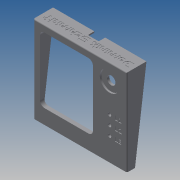
# Autodesk Inventor part: Top
Saved by Autodesk Inventor 2019 (Build 230136000, 136)
## iProperties
Created: 2022-10-27
Part Number: Top
Material: Generisch
Document SubType Name: Modeling
Designer: Dominik Schmidt
Density: 1 g/cm^3
Appearance: Vorgabe
Author: Dominik Schmidt
Autodesk Inventor part; units mm, degrees
ref_plane "YZ Plane" through (0, 0, 0) normal (1, 0, 0) x (0, 1, 0)
ref_plane "XZ Plane" through (0, 0, 0) normal (0, 1, 0) x (-1, 0, 0)
ref_plane "XY Plane" through (0, 0, 0) normal (0, 0, 1) x (1, 0, 0)
sketch "Skizze1" plane through (0, 0, 0) normal (0, 0, 1) x (1, 0, 0)
  line L0 (-19.1, 28.5) -> (19.1, 28.5)
  line L1 (23.1, 24.5) -> (23.1, -24.5)
  line L2 (19.1, -28.5) -> (-19.1, -28.5)
  line L3 (-23.1, -24.5) -> (-23.1, 24.5)
  line L4 (-23.1, 28.5) -> (23.1, -28.5) construction
  line L5 (23.1, 28.5) -> (-23.1, -28.5) construction
  circle A0 centre (37.5, 20) radius 3.7
  arc A1 (-19.1, 28.5) -> (-23.1, 24.5) centre (-19.1, 24.5) ccw
  arc A2 (23.1, 24.5) -> (19.1, 28.5) centre (19.1, 24.5) ccw
  arc A3 (-23.1, -24.5) -> (-19.1, -28.5) centre (-19.1, -24.5) ccw
  arc A4 (19.1, -28.5) -> (23.1, -24.5) centre (19.1, -24.5) ccw
  circle A5 centre (37.5, 20) radius 12
  line L6 (31.4, 28) -> (43.6, 28)
  line L7 (43.6, 28) -> (43.6, 12)
  line L8 (43.6, 12) -> (31.4, 12)
  line L9 (31.4, 12) -> (31.4, 28)
  line L10 (31.4, 28) -> (43.6, 12) construction
  line L11 (43.6, 28) -> (31.4, 12) construction
  line L12 (-25.5, 32) -> (25.5, 32)
  line L13 (25.5, 32) -> (25.5, -32)
  line L14 (25.5, -32) -> (-25.5, -32)
  line L15 (-25.5, -32) -> (-25.5, 32)
  line L16 (-25.5, 32) -> (25.5, -32) construction
  line L17 (25.5, 32) -> (-25.5, -32) construction
  circle A6 centre (37.5, -5) radius 1.5
  circle A7 centre (37.5, -13) radius 1.5
  circle A8 centre (37.5, -21) radius 1.5
  line L18 (-27.5, 33) -> (51.5, 33)
  line L19 (51.5, 33) -> (51.5, -33)
  line L20 (-27.5, -33) -> (-27.5, 33)
  line L21 (52.7, 34.2) -> (-28.7, 34.2)
  line L22 (-28.7, 34.2) -> (-28.7, -34.2)
  line L23 (52.7, -34.2) -> (52.7, 34.2)
  line L24 (-27.72, -34.2) -> (-27.2531, -34.2)
  line L25 (52.7, -34.2) -> (52.7, -41.2)
  line L26 (52.7, -41.2) -> (-28.7, -41.2)
  line L27 (-28.7, -41.2) -> (-28.7, -34.2)
  line L28 (-27.5, -33) -> (-27.5, -40)
  line L29 (-27.5, -40) -> (51.5, -40)
  line L30 (51.5, -40) -> (51.5, -33)
  point P0 (0, 0)
  dimension "d3" = 57
  dimension "d4" = 46.2
  dimension "d5" = 4
  dimension "d6" = 4
  dimension "d7" = 7.4
  dimension "d8" = 24
  dimension "d9" = 12.2
  dimension "d10" = 16
  dimension "d11" = 51
  dimension "d12" = 64
  dimension "d13" = 12
  dimension "d14" = 12
  dimension "d15" = 3
  dimension "d16" = 3
  dimension "d17" = 3
  dimension "d18" = 5
  dimension "d19" = 8
  dimension "d20" = 8
  dimension "d21" = 2
  dimension "d22" = 1
  dimension "d24" = 14
  dimension "d25" = 1.2
  dimension "d66" = 7
  dimension "d67" = 7
  constraints: 62 end point, 10 parallel, 10 point on line, 9 centre point, 9 perpendicular, 8 point on circle, 8 tangent, 6 midpoint, 4 horizontal, 2 equal radius, 1 coincident, 1 vertical, 1 other
  measures "d3" distance of L5.end L4.start
  measures "d4" distance of L4.start L5.start
  measures "d5" radius of A1
  measures "d6" radius of A2
  measures "d7" diameter of A0
  measures "d8" diameter of A5
  measures "d9" distance of L7.end L8.end
  measures "d10" distance of L6.end L7.end
  measures "d11" distance of L13.end L14.end
  measures "d12" distance of L12.end L13.end
  measures "d13" distance from line of L13 A0.centre
  measures "d14" distance from line of L12 A0.centre
  measures "d15" diameter of A6
  measures "d16" diameter of A7
  measures "d17" diameter of A8
  measures "d18" vertical distance of A6.centre point (0, 0)
  measures "d19" distance of A7.centre A6.centre
  measures "d20" distance of A8.centre A7.centre
  measures "d21" distance between parallel lines of L20 L15
  measures "d22" distance between parallel lines of L12 L18
  measures "d24" distance from line of L19 A0.centre
  measures "d25" distance between parallel lines of L18 L21
  measures "d66" distance of L23.start L25.end
  measures "d67" distance of L20.start L28.end
extrude "Extrusion1" add sketch "Skizze1" along normal blind 3.5 contours L13 L14 L15 L12
extrude "Extrusion2" add sketch "Skizze1" along normal blind 3.5 contours A5 | L6 L7 L8 L9 | L18 L19 L30 L29 L28 L20
extrude "Extrusion3" add sketch "Skizze1" along normal blind 3.5 and the other way blind 30 contours L23 L25 L26 L27 L22 L21
fillet "Rundung1" radius 1 3 edges at (-28.7, -3.5, 3.5) (12, 34.2, 3.5) (52.7, -3.5, 3.5)
sketch "Skizze2" plane through (0, 0, 3.5) normal (0, 0, 1) x (1, 0, 0)
  line L0 (33.8697, -1.9022) -> (41.4785, -1.9022)
  line L1 (41.4785, -1.9022) -> (41.4785, -24.9399)
  line L2 (41.4785, -24.9399) -> (33.8697, -24.9399)
  line L3 (33.8697, -24.9399) -> (33.8697, -1.9022)
  point P0 (0, 0)
  constraints: 8 end point, 2 parallel, 1 horizontal, 1 perpendicular
extrude "Extrusion4" add sketch "Skizze2" against normal blind 0.2
sketch "Skizze3" plane through (0, 0, 0) normal (0, 0, -1) x (-1, 0, 0)
  circle A0 centre (-37.5, -5) radius 1.5 projected
  circle A1 centre (-37.5, -5) radius 1.5
  circle A2 centre (-37.5, -13) radius 1.5 projected
  circle A3 centre (-37.5, -13) radius 1.5
  circle A4 centre (-37.5, -21) radius 1.5 projected
  circle A5 centre (-37.5, -21) radius 1.5
  circle A6 centre (-37.5, -5) radius 2.5
  circle A7 centre (-37.5, -13) radius 2.5
  circle A8 centre (-37.5, -21) radius 2.5
  point P0 (0, 0)
  dimension "d37" = 3
  dimension "d38" = 3
  dimension "d39" = 5
  dimension "d40" = 5
  dimension "d41" = 5
  constraints: 6 centre point, 6 coincident
  measures "d37" diameter of A1
  measures "d38" diameter of A3
  measures "d39" diameter of A6
  measures "d40" diameter of A7
  measures "d41" diameter of A8
extrude "Extrusion5" add sketch "Skizze3" along normal blind 1
sketch "Skizze4" plane through (52.7, -34.2, -30) normal (1, 0, 0) x (0, 0, -1)
  line L0 (-32.5, 68.4) -> (0, 68.4) projected
  line L1 (-32.5, 68.4) -> (-32.5, 0)
  line L2 (-32.5, 68.4) -> (-16.5, 68.4)
  line L3 (0, 68.4) -> (0, -7) projected
  line L4 (0, 0) -> (0, 68.4)
  line L5 (-32.5, -7) -> (-32.5, 68.4) projected
  line L6 (-32.5, 0) -> (-32.5, -7)
  line L7 (-32.5, -7) -> (-26.5, -7)
  line L8 (-26.5, -7) -> (-16.5, 68.4)
  line L9 (0, -7) -> (-32.5, -7) projected
  line L10 (-26.5, -7) -> (0, -7)
  point P0 (-30, 34.2)
  dimension "d45" = 16
  dimension "d68" = 6
  constraints: 14 end point, 2 collinear, 1 perpendicular, 1 point on line
  measures "d45" distance of L0.start L2.end
  measures "d68" distance of L5.start L7.end
sketch "Skizze6" plane through (-28.7, 34.2, 2.5) normal (0, 1, 0) x (1, 0, 0)
  line L0 (78.4875, 2.7744) -> (3.0019, 2.7744) construction
  line L1 (3.0019, 2.7744) -> (3.0019, 8.8744) construction
  line L2 (3.0019, 8.8744) -> (78.4875, 8.8744) construction
  line L3 (78.4875, 8.8744) -> (78.4875, 2.7744) construction
  spline S0 degree 2 poles (72.0827, 5.8217) (72.0827, 7.0827) (72.9812, 7.9812) knots 0 0 0 1 1 1
  spline S1 degree 2 poles (72.9812, 7.9812) (73.8744, 8.8744) (75.1406, 8.8744) knots 0 0 0 1 1 1
  line L4 (75.1406, 8.8744) -> (78.188, 8.8744)
  line L5 (78.188, 8.8744) -> (78.188, 7.5293)
  line L6 (78.188, 7.5293) -> (75.1406, 7.5293)
  spline S2 degree 2 poles (75.1406, 7.5293) (74.4418, 7.5293) (73.9374, 7.0302) knots 0 0 0 1 1 1
  spline S3 degree 2 poles (73.9374, 7.0302) (73.433, 6.5205) (73.433, 5.8217) knots 0 0 0 1 1 1
  spline S4 degree 2 poles (73.433, 5.8217) (73.433, 5.123) (73.9374, 4.6238) knots 0 0 0 1 1 1
  spline S5 degree 2 poles (73.9374, 4.6238) (74.4366, 4.1194) (75.1406, 4.1194) knots 0 0 0 1 1 1
  line L7 (75.1406, 4.1194) -> (78.188, 4.1194)
  line L8 (78.188, 4.1194) -> (78.188, 2.7744)
  line L9 (78.188, 2.7744) -> (75.1406, 2.7744)
  spline S6 degree 2 poles (75.1406, 2.7744) (73.8744, 2.7744) (72.9812, 3.6728) knots 0 0 0 1 1 1
  spline S7 degree 2 poles (72.9812, 3.6728) (72.0827, 4.5713) (72.0827, 5.8217) knots 0 0 0 1 1 1
  spline S8 degree 2 poles (74.4576, 5.8217) (74.4576, 6.1002) (74.6625, 6.2999) knots 0 0 0 1 1 1
  spline S9 degree 2 poles (74.6625, 6.2999) (74.8569, 6.4943) (75.1406, 6.4943) knots 0 0 0 1 1 1
  spline S10 degree 2 poles (75.1406, 6.4943) (75.4138, 6.4943) (75.6135, 6.2946) knots 0 0 0 1 1 1
  spline S11 degree 2 poles (75.6135, 6.2946) (75.8131, 6.0897) (75.8131, 5.8217) knots 0 0 0 1 1 1
  spline S12 degree 2 poles (75.8131, 5.8217) (75.8131, 5.5485) (75.4138, 5.1492) (75.1406, 5.1492) knots 0 0 0 1 2 2 2
  spline S13 degree 2 poles (75.1406, 5.1492) (74.8622, 5.1492) (74.4576, 5.5538) (74.4576, 5.8217) knots 0 0 0 1 2 2 2
  spline S14 degree 2 poles (66.8917, 6.4155) (66.8917, 7.4242) (68.3418, 8.8744) (69.3559, 8.8744) knots 0 0 0 1 2 2 2
  spline S15 degree 2 poles (69.3559, 8.8744) (70.3647, 8.8744) (71.8148, 7.4242) (71.8148, 6.4155) knots 0 0 0 1 2 2 2
  spline S16 degree 2 poles (71.8148, 6.4155) (71.8148, 5.4067) (71.0897, 4.6869) knots 0 0 0 1 1 1
  spline S17 degree 2 poles (71.0897, 4.6869) (70.3647, 3.9618) (69.3559, 3.9618) knots 0 0 0 1 1 1
  spline S18 degree 2 poles (69.3559, 3.9618) (68.3418, 3.9618) (67.6168, 4.6869) knots 0 0 0 1 1 1
  spline S19 degree 2 poles (67.6168, 4.6869) (66.8917, 5.4119) (66.8917, 6.4155) knots 0 0 0 1 1 1
  spline S20 degree 2 poles (68.242, 6.4155) (68.242, 5.9689) (68.5993, 5.5223) knots 0 0 0 1 1 1
  spline S21 degree 2 poles (68.5993, 5.5223) (68.9093, 5.3068) (69.3559, 5.3068) knots 0 0 0 1 1 1
  spline S22 degree 2 poles (69.3559, 5.3068) (69.8025, 5.3068) (70.1335, 5.6379) knots 0 0 0 1 1 1
  spline S23 degree 2 poles (70.1335, 5.6379) (70.4645, 5.9689) (70.4645, 6.4155) knots 0 0 0 1 1 1
  spline S24 degree 2 poles (70.4645, 6.4155) (70.4645, 6.8673) (69.8025, 7.5293) (69.3559, 7.5293) knots 0 0 0 1 2 2 2
  spline S25 degree 2 poles (69.3559, 7.5293) (68.9093, 7.5293) (68.242, 6.8621) (68.242, 6.4155) knots 0 0 0 1 2 2 2
  spline S26 degree 2 poles (68.6781, 6.4155) (68.6781, 6.6887) (69.0774, 7.088) (69.3559, 7.088) knots 0 0 0 1 2 2 2
  spline S27 degree 2 poles (69.3559, 7.088) (69.6396, 7.088) (70.0284, 6.6992) (70.0284, 6.4155) knots 0 0 0 1 2 2 2
  spline S28 degree 2 poles (70.0284, 6.4155) (70.0284, 6.1475) (69.8287, 5.9478) knots 0 0 0 1 1 1
  spline S29 degree 2 poles (69.8287, 5.9478) (69.6238, 5.7429) (69.3559, 5.7429) knots 0 0 0 1 1 1
  spline S30 degree 2 poles (69.3559, 5.7429) (69.0827, 5.7429) (68.9408, 5.9216) knots 0 0 0 1 1 1
  spline S31 degree 2 poles (68.9408, 5.9216) (68.6781, 6.1475) (68.6781, 6.4155) knots 0 0 0 1 1 1
  line L10 (58.0228, 8.8744) -> (59.3731, 8.8744)
  line L11 (59.3731, 8.8744) -> (59.3731, 6.4155)
  spline S32 degree 2 poles (59.3731, 6.4155) (59.3731, 5.9689) (59.6463, 5.6641) knots 0 0 0 1 1 1
  spline S33 degree 2 poles (59.6463, 5.6641) (60.0351, 5.3068) (60.4817, 5.3068) knots 0 0 0 1 1 1
  spline S34 degree 2 poles (60.4817, 5.3068) (60.9231, 5.3068) (61.2541, 5.6379) knots 0 0 0 1 1 1
  spline S35 degree 2 poles (61.2541, 5.6379) (61.5851, 5.9636) (61.5851, 6.4155) knots 0 0 0 1 1 1
  line L12 (61.5851, 6.4155) -> (61.5851, 8.8744)
  line L13 (61.5851, 8.8744) -> (62.9354, 8.8744)
  line L14 (62.9354, 8.8744) -> (62.9354, 6.4155)
  spline S36 degree 2 poles (62.9354, 6.4155) (62.9354, 5.9689) (63.2926, 5.5801) knots 0 0 0 1 1 1
  spline S37 degree 2 poles (63.2926, 5.5801) (63.5974, 5.3068) (64.044, 5.3068) knots 0 0 0 1 1 1
  spline S38 degree 2 poles (64.044, 5.3068) (64.4906, 5.3068) (64.8268, 5.6379) knots 0 0 0 1 1 1
  spline S39 degree 2 poles (64.8268, 5.6379) (65.1526, 5.9636) (65.1526, 6.4155) knots 0 0 0 1 1 1
  line L15 (65.1526, 6.4155) -> (65.1526, 8.8744)
  line L16 (65.1526, 8.8744) -> (66.5029, 8.8744)
  line L17 (66.5029, 8.8744) -> (66.5029, 3.9618)
  line L18 (66.5029, 3.9618) -> (65.1526, 3.9618)
  line L19 (65.1526, 3.9618) -> (65.1526, 4.2823)
  spline S40 degree 2 poles (65.1526, 4.2823) (64.7113, 3.9618) (64.0492, 3.9618) knots 0 0 0 1 1 1
  spline S41 degree 2 poles (64.0492, 3.9618) (62.9406, 3.9618) (62.2628, 4.7709) knots 0 0 0 1 1 1
  spline S42 degree 2 poles (62.2628, 4.7709) (61.5798, 3.9618) (60.4817, 3.9618) knots 0 0 0 1 1 1
  spline S43 degree 2 poles (60.4817, 3.9618) (59.4729, 3.9618) (58.7479, 4.6869) knots 0 0 0 1 1 1
  spline S44 degree 2 poles (58.7479, 4.6869) (58.0228, 5.4119) (58.0228, 6.4155) knots 0 0 0 1 1 1
  line L20 (58.0228, 6.4155) -> (58.0228, 8.8744)
  spline S45 degree 2 poles (59.8039, 6.4155) (59.8039, 6.6782) (60.2085, 7.088) (60.4817, 7.088) knots 0 0 0 1 2 2 2
  spline S46 degree 2 poles (60.4817, 7.088) (60.7549, 7.088) (61.1542, 6.6887) (61.1542, 6.4155) knots 0 0 0 1 2 2 2
  spline S47 degree 2 poles (61.1542, 6.4155) (61.1542, 6.1475) (60.9546, 5.9478) knots 0 0 0 1 1 1
  spline S48 degree 2 poles (60.9546, 5.9478) (60.7549, 5.7429) (60.4817, 5.7429) knots 0 0 0 1 1 1
  spline S49 degree 2 poles (60.4817, 5.7429) (60.2085, 5.7429) (60.0088, 5.9478) knots 0 0 0 1 1 1
  spline S50 degree 2 poles (60.0088, 5.9478) (59.8039, 6.1475) (59.8039, 6.4155) knots 0 0 0 1 1 1
  spline S51 degree 2 poles (63.3715, 6.4155) (63.3715, 6.6782) (63.7813, 7.088) (64.0492, 7.088) knots 0 0 0 1 2 2 2
  spline S52 degree 2 poles (64.0492, 7.088) (64.3172, 7.088) (64.5221, 6.8883) knots 0 0 0 1 1 1
  spline S53 degree 2 poles (64.5221, 6.8883) (64.7218, 6.6887) (64.7218, 6.4155) knots 0 0 0 1 1 1
  spline S54 degree 2 poles (64.7218, 6.4155) (64.7218, 6.1475) (64.5221, 5.9478) knots 0 0 0 1 1 1
  spline S55 degree 2 poles (64.5221, 5.9478) (64.3172, 5.7429) (64.0492, 5.7429) knots 0 0 0 1 1 1
  spline S56 degree 2 poles (64.0492, 5.7429) (63.776, 5.7429) (63.6342, 5.9216) knots 0 0 0 1 1 1
  spline S57 degree 2 poles (63.6342, 5.9216) (63.3715, 6.1475) (63.3715, 6.4155) knots 0 0 0 1 1 1
  line L21 (56.0525, 8.8744) -> (57.4028, 8.8744)
  line L22 (57.4028, 8.8744) -> (57.4028, 5.7429)
  line L23 (57.4028, 5.7429) -> (56.0525, 5.7429)
  line L24 (56.0525, 5.7429) -> (56.0525, 8.8744)
  spline S58 degree 2 poles (56.0525, 4.6343) (56.0525, 4.9023) (56.2574, 5.1072) knots 0 0 0 1 1 1
  spline S59 degree 2 poles (56.2574, 5.1072) (56.4571, 5.3068) (56.7303, 5.3068) knots 0 0 0 1 1 1
  spline S60 degree 2 poles (56.7303, 5.3068) (57.0035, 5.3068) (57.2032, 5.1072) knots 0 0 0 1 1 1
  spline S61 degree 2 poles (57.2032, 5.1072) (57.4028, 4.9023) (57.4028, 4.6343) knots 0 0 0 1 1 1
  spline S62 degree 2 poles (57.4028, 4.6343) (57.4028, 4.3611) (57.0035, 3.9618) (56.7303, 3.9618) knots 0 0 0 1 2 2 2
  spline S63 degree 2 poles (56.7303, 3.9618) (56.4571, 3.9618) (56.0525, 4.3664) (56.0525, 4.6343) knots 0 0 0 1 2 2 2
  line L25 (50.6566, 8.8744) -> (52.0069, 8.8744)
  line L26 (52.0069, 8.8744) -> (52.0069, 6.4155)
  spline S64 degree 2 poles (52.0069, 6.4155) (52.0069, 5.9689) (52.3641, 5.5801) knots 0 0 0 1 1 1
  spline S65 degree 2 poles (52.3641, 5.5801) (52.6689, 5.3068) (53.1155, 5.3068) knots 0 0 0 1 1 1
  spline S66 degree 2 poles (53.1155, 5.3068) (53.5621, 5.3068) (53.8983, 5.6379) knots 0 0 0 1 1 1
  spline S67 degree 2 poles (53.8983, 5.6379) (54.2241, 5.9636) (54.2241, 6.4155) knots 0 0 0 1 1 1
  line L27 (54.2241, 6.4155) -> (54.2241, 8.8744)
  line L28 (54.2241, 8.8744) -> (55.5744, 8.8744)
  line L29 (55.5744, 8.8744) -> (55.5744, 3.9618)
  line L30 (55.5744, 3.9618) -> (54.2241, 3.9618)
  line L31 (54.2241, 3.9618) -> (54.2241, 4.2823)
  spline S68 degree 2 poles (54.2241, 4.2823) (53.7827, 3.9618) (53.1207, 3.9618) knots 0 0 0 1 1 1
  spline S69 degree 2 poles (53.1207, 3.9618) (52.1067, 3.9618) (51.3816, 4.6869) knots 0 0 0 1 1 1
  spline S70 degree 2 poles (51.3816, 4.6869) (50.6566, 5.4119) (50.6566, 6.4155) knots 0 0 0 1 1 1
  line L32 (50.6566, 6.4155) -> (50.6566, 8.8744)
  spline S71 degree 2 poles (52.4429, 6.4155) (52.4429, 6.6887) (52.8423, 7.088) (53.1207, 7.088) knots 0 0 0 1 2 2 2
  spline S72 degree 2 poles (53.1207, 7.088) (53.3887, 7.088) (53.5936, 6.8936) knots 0 0 0 1 1 1
  spline S73 degree 2 poles (53.5936, 6.8936) (53.7932, 6.6887) (53.7932, 6.4155) knots 0 0 0 1 1 1
  spline S74 degree 2 poles (53.7932, 6.4155) (53.7932, 6.137) (53.5988, 5.9426) knots 0 0 0 1 1 1
  spline S75 degree 2 poles (53.5988, 5.9426) (53.3992, 5.7429) (53.1207, 5.7429) knots 0 0 0 1 1 1
  spline S76 degree 2 poles (53.1207, 5.7429) (52.8475, 5.7429) (52.7057, 5.9216) knots 0 0 0 1 1 1
  spline S77 degree 2 poles (52.7057, 5.9216) (52.4429, 6.1475) (52.4429, 6.4155) knots 0 0 0 1 1 1
  line L33 (48.7598, 8.8744) -> (50.1101, 8.8744)
  line L34 (50.1101, 8.8744) -> (50.1101, 5.7429)
  line L35 (50.1101, 5.7429) -> (48.7598, 5.7429)
  line L36 (48.7598, 5.7429) -> (48.7598, 8.8744)
  spline S78 degree 2 poles (48.7598, 4.6343) (48.7598, 4.9023) (48.9647, 5.1072) knots 0 0 0 1 1 1
  spline S79 degree 2 poles (48.9647, 5.1072) (49.1644, 5.3068) (49.4376, 5.3068) knots 0 0 0 1 1 1
  spline S80 degree 2 poles (49.4376, 5.3068) (49.7108, 5.3068) (49.9105, 5.1072) knots 0 0 0 1 1 1
  spline S81 degree 2 poles (49.9105, 5.1072) (50.1101, 4.9023) (50.1101, 4.6343) knots 0 0 0 1 1 1
  spline S82 degree 2 poles (50.1101, 4.6343) (50.1101, 4.3611) (49.7108, 3.9618) (49.4376, 3.9618) knots 0 0 0 1 2 2 2
  spline S83 degree 2 poles (49.4376, 3.9618) (49.1644, 3.9618) (48.7598, 4.3664) (48.7598, 4.6343) knots 0 0 0 1 2 2 2
  line L37 (43.3639, 8.8744) -> (44.7142, 8.8744)
  line L38 (44.7142, 8.8744) -> (44.7142, 7.6081)
  spline S84 degree 2 poles (44.7142, 7.6081) (44.7142, 7.1563) (45.0715, 6.7727) knots 0 0 0 1 1 1
  spline S85 degree 2 poles (45.0715, 6.7727) (45.3762, 6.4943) (45.8228, 6.4943) knots 0 0 0 1 1 1
  spline S86 degree 2 poles (45.8228, 6.4943) (46.2694, 6.4943) (46.6057, 6.8305) knots 0 0 0 1 1 1
  spline S87 degree 2 poles (46.6057, 6.8305) (46.9314, 7.1563) (46.9314, 7.6081) knots 0 0 0 1 1 1
  line L39 (46.9314, 7.6081) -> (46.9314, 8.8744)
  line L40 (46.9314, 8.8744) -> (48.2817, 8.8744)
  line L41 (48.2817, 8.8744) -> (48.2817, 2.7744)
  line L42 (48.2817, 2.7744) -> (46.9314, 2.7744)
  line L43 (46.9314, 2.7744) -> (46.9314, 5.4697)
  line L44 (46.9314, 5.4697) -> (45.8648, 3.9618)
  line L45 (45.8648, 3.9618) -> (44.2571, 3.9618)
  line L46 (44.2571, 3.9618) -> (45.2343, 5.2333)
  spline S88 degree 2 poles (45.2343, 5.2333) (44.4567, 5.3909) (44.0574, 6.0372) knots 0 0 0 1 1 1
  spline S89 degree 2 poles (44.0574, 6.0372) (43.3639, 6.7517) (43.3639, 7.6081) knots 0 0 0 1 1 1
  line L47 (43.3639, 7.6081) -> (43.3639, 8.8744)
  spline S90 degree 2 poles (45.1503, 7.6081) (45.1503, 7.8761) (45.5496, 8.2807) (45.828, 8.2807) knots 0 0 0 1 2 2 2
  spline S91 degree 2 poles (45.828, 8.2807) (46.096, 8.2807) (46.5006, 7.8708) (46.5006, 7.6081) knots 0 0 0 1 2 2 2
  spline S92 degree 2 poles (46.5006, 7.6081) (46.5006, 7.3349) (46.3009, 7.1353) knots 0 0 0 1 1 1
  spline S93 degree 2 poles (46.3009, 7.1353) (46.096, 6.9304) (45.828, 6.9304) knots 0 0 0 1 1 1
  spline S94 degree 2 poles (45.828, 6.9304) (45.5548, 6.9304) (45.413, 7.1143) knots 0 0 0 1 1 1
  spline S95 degree 2 poles (45.413, 7.1143) (45.1503, 7.3402) (45.1503, 7.6081) knots 0 0 0 1 1 1
  line L48 (34.5843, 4.1194) -> (38.8296, 4.1194)
  spline S96 degree 2 poles (38.8296, 4.1194) (39.0345, 4.1194) (39.1921, 4.2718) knots 0 0 0 1 1 1
  spline S97 degree 2 poles (39.1921, 4.2718) (39.3392, 4.4242) (39.3392, 4.6343) knots 0 0 0 1 1 1
  spline S98 degree 2 poles (39.3392, 4.6343) (39.3392, 4.8497) (39.0398, 5.1492) (38.7455, 5.1492) knots 0 0 0 1 2 2 2
  line L49 (38.7455, 5.1492) -> (38.7455, 6.4943)
  spline S99 degree 2 poles (38.7455, 6.4943) (39.5967, 6.4943) (40.1431, 5.9531) knots 0 0 0 1 1 1
  spline S100 degree 2 poles (40.1431, 5.9531) (40.6895, 5.4067) (40.6895, 4.6343) knots 0 0 0 1 1 1
  spline S101 degree 2 poles (40.6895, 4.6343) (40.6895, 3.862) (40.1484, 3.3208) knots 0 0 0 1 1 1
  spline S102 degree 2 poles (40.1484, 3.3208) (39.6019, 2.7744) (38.8296, 2.7744) knots 0 0 0 1 1 1
  line L50 (38.8296, 2.7744) -> (34.5843, 2.7744)
  line L51 (34.5843, 2.7744) -> (34.5843, 4.1194)
  spline S103 degree 2 poles (34.5843, 7.0092) (34.5843, 7.7815) (35.136, 8.3332) knots 0 0 0 1 1 1
  spline S104 degree 2 poles (35.136, 8.3332) (35.6771, 8.8744) (36.4495, 8.8744) knots 0 0 0 1 1 1
  line L52 (36.4495, 8.8744) -> (40.6895, 8.8744)
  line L53 (40.6895, 8.8744) -> (40.6895, 7.5293)
  line L54 (40.6895, 7.5293) -> (36.4495, 7.5293)
  spline S105 degree 2 poles (36.4495, 7.5293) (36.2393, 7.5293) (36.0922, 7.377) knots 0 0 0 1 1 1
  spline S106 degree 2 poles (36.0922, 7.377) (35.9346, 7.2246) (35.9346, 7.0092) knots 0 0 0 1 1 1
  spline S107 degree 2 poles (35.9346, 7.0092) (35.9346, 6.8043) (36.1132, 6.5941) knots 0 0 0 1 1 1
  spline S108 degree 2 poles (36.1132, 6.5941) (36.2393, 6.4995) (36.5283, 6.4943) knots 0 0 0 1 1 1
  line L55 (36.5283, 6.4943) -> (36.5283, 5.1492)
  spline S109 degree 2 poles (36.5283, 5.1492) (35.6771, 5.1492) (35.136, 5.6956) knots 0 0 0 1 1 1
  spline S110 degree 2 poles (35.136, 5.6956) (34.5843, 6.2421) (34.5843, 7.0092) knots 0 0 0 1 1 1
  spline S111 degree 2 poles (36.9591, 5.8217) (36.9591, 6.095) (37.1641, 6.2999) knots 0 0 0 1 1 1
  spline S112 degree 2 poles (37.1641, 6.2999) (37.3585, 6.4943) (37.6422, 6.4943) knots 0 0 0 1 1 1
  spline S113 degree 2 poles (37.6422, 6.4943) (37.9206, 6.4943) (38.3147, 6.1055) (38.3147, 5.8217) knots 0 0 0 1 2 2 2
  spline S114 degree 2 poles (38.3147, 5.8217) (38.3147, 5.5485) (37.9154, 5.1492) (37.6422, 5.1492) knots 0 0 0 1 2 2 2
  spline S115 degree 2 poles (37.6422, 5.1492) (37.369, 5.1492) (37.143, 5.4119) knots 0 0 0 1 1 1
  spline S116 degree 2 poles (37.143, 5.4119) (36.9591, 5.5538) (36.9591, 5.8217) knots 0 0 0 1 1 1
  spline S117 degree 2 poles (29.9449, 8.0968) (30.6963, 8.8744) (31.705, 8.8744) knots 0 0 0 1 1 1
  spline S118 degree 2 poles (31.705, 8.8744) (32.7191, 8.8744) (34.164, 7.4242) (34.164, 6.4155) knots 0 0 0 1 2 2 2
  spline S119 degree 2 poles (34.164, 6.4155) (34.164, 5.4067) (33.4389, 4.6869) knots 0 0 0 1 1 1
  spline S120 degree 2 poles (33.4389, 4.6869) (32.7138, 3.9618) (31.705, 3.9618) knots 0 0 0 1 1 1
  spline S121 degree 2 poles (31.705, 3.9618) (30.6963, 3.9618) (29.9449, 4.7447) knots 0 0 0 1 1 1
  line L56 (29.9449, 4.7447) -> (30.8644, 5.6589)
  spline S122 degree 2 poles (30.8644, 5.6589) (31.2585, 5.3068) (31.705, 5.3068) knots 0 0 0 1 1 1
  spline S123 degree 2 poles (31.705, 5.3068) (32.1516, 5.3068) (32.4827, 5.6379) knots 0 0 0 1 1 1
  spline S124 degree 2 poles (32.4827, 5.6379) (32.8137, 5.9689) (32.8137, 6.4155) knots 0 0 0 1 1 1
  spline S125 degree 2 poles (32.8137, 6.4155) (32.8137, 6.8673) (32.1516, 7.5293) (31.705, 7.5293) knots 0 0 0 1 2 2 2
  spline S126 degree 2 poles (31.705, 7.5293) (31.2585, 7.5293) (30.8644, 7.1773) knots 0 0 0 1 1 1
  line L57 (30.8644, 7.1773) -> (29.9449, 8.0968)
  spline S127 degree 2 poles (31.0273, 6.4155) (31.0273, 6.6887) (31.4266, 7.088) (31.705, 7.088) knots 0 0 0 1 2 2 2
  spline S128 degree 2 poles (31.705, 7.088) (31.9888, 7.088) (32.3776, 6.6992) (32.3776, 6.4155) knots 0 0 0 1 2 2 2
  spline S129 degree 2 poles (32.3776, 6.4155) (32.3776, 6.1475) (32.1779, 5.9478) knots 0 0 0 1 1 1
  spline S130 degree 2 poles (32.1779, 5.9478) (31.973, 5.7429) (31.705, 5.7429) knots 0 0 0 1 1 1
  spline S131 degree 2 poles (31.705, 5.7429) (31.4318, 5.7429) (31.29, 5.9216) knots 0 0 0 1 1 1
  spline S132 degree 2 poles (31.29, 5.9216) (31.0273, 6.1475) (31.0273, 6.4155) knots 0 0 0 1 1 1
  line L58 (24.6488, 8.8744) -> (25.9991, 8.8744)
  line L59 (25.9991, 8.8744) -> (25.9991, 6.4155)
  spline S133 degree 2 poles (25.9991, 6.4155) (25.9991, 5.9689) (26.3564, 5.5801) knots 0 0 0 1 1 1
  spline S134 degree 2 poles (26.3564, 5.5801) (26.6611, 5.3068) (27.1077, 5.3068) knots 0 0 0 1 1 1
  spline S135 degree 2 poles (27.1077, 5.3068) (27.5543, 5.3068) (27.8906, 5.6379) knots 0 0 0 1 1 1
  spline S136 degree 2 poles (27.8906, 5.6379) (28.2163, 5.9636) (28.2163, 6.4155) knots 0 0 0 1 1 1
  line L60 (28.2163, 6.4155) -> (28.2163, 8.8744)
  line L61 (28.2163, 8.8744) -> (29.5666, 8.8744)
  line L62 (29.5666, 8.8744) -> (29.5666, 2.7744)
  line L63 (29.5666, 2.7744) -> (28.2163, 2.7744)
  line L64 (28.2163, 2.7744) -> (28.2163, 4.2823)
  spline S137 degree 2 poles (28.2163, 4.2823) (27.775, 3.9618) (27.113, 3.9618) knots 0 0 0 1 1 1
  spline S138 degree 2 poles (27.113, 3.9618) (26.0989, 3.9618) (25.3739, 4.6869) knots 0 0 0 1 1 1
  spline S139 degree 2 poles (25.3739, 4.6869) (24.6488, 5.4119) (24.6488, 6.4155) knots 0 0 0 1 1 1
  line L65 (24.6488, 6.4155) -> (24.6488, 8.8744)
  spline S140 degree 2 poles (26.4352, 6.4155) (26.4352, 6.6887) (26.8345, 7.088) (27.113, 7.088) knots 0 0 0 1 2 2 2
  spline S141 degree 2 poles (27.113, 7.088) (27.3809, 7.088) (27.5858, 6.8936) knots 0 0 0 1 1 1
  spline S142 degree 2 poles (27.5858, 6.8936) (27.7855, 6.6887) (27.7855, 6.4155) knots 0 0 0 1 1 1
  spline S143 degree 2 poles (27.7855, 6.4155) (27.7855, 6.1475) (27.5858, 5.9478) knots 0 0 0 1 1 1
  spline S144 degree 2 poles (27.5858, 5.9478) (27.3809, 5.7429) (27.113, 5.7429) knots 0 0 0 1 1 1
  spline S145 degree 2 poles (27.113, 5.7429) (26.8345, 5.7429) (26.6349, 5.9426) knots 0 0 0 1 1 1
  spline S146 degree 2 poles (26.6349, 5.9426) (26.4352, 6.1422) (26.4352, 6.4155) knots 0 0 0 1 1 1
  line L66 (15.6223, 8.8744) -> (16.9726, 8.8744)
  line L67 (16.9726, 8.8744) -> (16.9726, 6.4155)
  spline S147 degree 2 poles (16.9726, 6.4155) (16.9726, 5.9689) (17.2458, 5.6641) knots 0 0 0 1 1 1
  spline S148 degree 2 poles (17.2458, 5.6641) (17.6346, 5.3068) (18.0812, 5.3068) knots 0 0 0 1 1 1
  spline S149 degree 2 poles (18.0812, 5.3068) (18.5225, 5.3068) (18.8535, 5.6379) knots 0 0 0 1 1 1
  spline S150 degree 2 poles (18.8535, 5.6379) (19.1845, 5.9636) (19.1845, 6.4155) knots 0 0 0 1 1 1
  line L68 (19.1845, 6.4155) -> (19.1845, 8.8744)
  line L69 (19.1845, 8.8744) -> (20.5349, 8.8744)
  line L70 (20.5349, 8.8744) -> (20.5349, 6.4155)
  spline S151 degree 2 poles (20.5349, 6.4155) (20.5349, 5.9689) (20.8921, 5.5801) knots 0 0 0 1 1 1
  spline S152 degree 2 poles (20.8921, 5.5801) (21.1969, 5.3068) (21.6435, 5.3068) knots 0 0 0 1 1 1
  spline S153 degree 2 poles (21.6435, 5.3068) (22.0901, 5.3068) (22.4263, 5.6379) knots 0 0 0 1 1 1
  spline S154 degree 2 poles (22.4263, 5.6379) (22.7521, 5.9636) (22.7521, 6.4155) knots 0 0 0 1 1 1
  line L71 (22.7521, 6.4155) -> (22.7521, 8.8744)
  line L72 (22.7521, 8.8744) -> (24.1024, 8.8744)
  line L73 (24.1024, 8.8744) -> (24.1024, 3.9618)
  line L74 (24.1024, 3.9618) -> (22.7521, 3.9618)
  line L75 (22.7521, 3.9618) -> (22.7521, 4.2823)
  spline S155 degree 2 poles (22.7521, 4.2823) (22.3107, 3.9618) (21.6487, 3.9618) knots 0 0 0 1 1 1
  spline S156 degree 2 poles (21.6487, 3.9618) (20.5401, 3.9618) (19.8623, 4.7709) knots 0 0 0 1 1 1
  spline S157 degree 2 poles (19.8623, 4.7709) (19.1793, 3.9618) (18.0812, 3.9618) knots 0 0 0 1 1 1
  spline S158 degree 2 poles (18.0812, 3.9618) (17.0724, 3.9618) (16.3473, 4.6869) knots 0 0 0 1 1 1
  spline S159 degree 2 poles (16.3473, 4.6869) (15.6223, 5.4119) (15.6223, 6.4155) knots 0 0 0 1 1 1
  line L76 (15.6223, 6.4155) -> (15.6223, 8.8744)
  spline S160 degree 2 poles (17.4034, 6.4155) (17.4034, 6.6782) (17.808, 7.088) (18.0812, 7.088) knots 0 0 0 1 2 2 2
  spline S161 degree 2 poles (18.0812, 7.088) (18.3544, 7.088) (18.7537, 6.6887) (18.7537, 6.4155) knots 0 0 0 1 2 2 2
  spline S162 degree 2 poles (18.7537, 6.4155) (18.7537, 6.1475) (18.5541, 5.9478) knots 0 0 0 1 1 1
  spline S163 degree 2 poles (18.5541, 5.9478) (18.3544, 5.7429) (18.0812, 5.7429) knots 0 0 0 1 1 1
  spline S164 degree 2 poles (18.0812, 5.7429) (17.808, 5.7429) (17.6083, 5.9478) knots 0 0 0 1 1 1
  spline S165 degree 2 poles (17.6083, 5.9478) (17.4034, 6.1475) (17.4034, 6.4155) knots 0 0 0 1 1 1
  spline S166 degree 2 poles (20.9709, 6.4155) (20.9709, 6.6782) (21.3808, 7.088) (21.6487, 7.088) knots 0 0 0 1 2 2 2
  spline S167 degree 2 poles (21.6487, 7.088) (21.9167, 7.088) (22.1216, 6.8883) knots 0 0 0 1 1 1
  spline S168 degree 2 poles (22.1216, 6.8883) (22.3212, 6.6887) (22.3212, 6.4155) knots 0 0 0 1 1 1
  spline S169 degree 2 poles (22.3212, 6.4155) (22.3212, 6.1475) (22.1216, 5.9478) knots 0 0 0 1 1 1
  spline S170 degree 2 poles (22.1216, 5.9478) (21.9167, 5.7429) (21.6487, 5.7429) knots 0 0 0 1 1 1
  spline S171 degree 2 poles (21.6487, 5.7429) (21.3755, 5.7429) (21.2336, 5.9216) knots 0 0 0 1 1 1
  spline S172 degree 2 poles (21.2336, 5.9216) (20.9709, 6.1475) (20.9709, 6.4155) knots 0 0 0 1 1 1
  line L77 (13.652, 8.8744) -> (15.0023, 8.8744)
  line L78 (15.0023, 8.8744) -> (15.0023, 5.7429)
  line L79 (15.0023, 5.7429) -> (13.652, 5.7429)
  line L80 (13.652, 5.7429) -> (13.652, 8.8744)
  spline S173 degree 2 poles (13.652, 4.6343) (13.652, 4.9023) (13.8569, 5.1072) knots 0 0 0 1 1 1
  spline S174 degree 2 poles (13.8569, 5.1072) (14.0566, 5.3068) (14.3298, 5.3068) knots 0 0 0 1 1 1
  spline S175 degree 2 poles (14.3298, 5.3068) (14.603, 5.3068) (14.8026, 5.1072) knots 0 0 0 1 1 1
  spline S176 degree 2 poles (14.8026, 5.1072) (15.0023, 4.9023) (15.0023, 4.6343) knots 0 0 0 1 1 1
  spline S177 degree 2 poles (15.0023, 4.6343) (15.0023, 4.3611) (14.603, 3.9618) (14.3298, 3.9618) knots 0 0 0 1 2 2 2
  spline S178 degree 2 poles (14.3298, 3.9618) (14.0566, 3.9618) (13.652, 4.3664) (13.652, 4.6343) knots 0 0 0 1 2 2 2
  line L81 (8.4032, 8.8744) -> (9.7535, 8.8744)
  line L82 (9.7535, 8.8744) -> (9.7535, 8.5539)
  spline S179 degree 2 poles (9.7535, 8.5539) (10.2001, 8.8744) (10.8621, 8.8744) knots 0 0 0 1 1 1
  spline S180 degree 2 poles (10.8621, 8.8744) (11.8761, 8.8744) (13.3262, 7.4242) (13.3262, 6.4155) knots 0 0 0 1 2 2 2
  spline S181 degree 2 poles (13.3262, 6.4155) (13.3262, 5.4067) (12.6012, 4.6869) knots 0 0 0 1 1 1
  spline S182 degree 2 poles (12.6012, 4.6869) (11.8761, 3.9618) (10.8621, 3.9618) knots 0 0 0 1 1 1
  spline S183 degree 2 poles (10.8621, 3.9618) (10.2106, 3.9618) (9.7535, 4.2823) knots 0 0 0 1 1 1
  line L83 (9.7535, 4.2823) -> (9.7535, 2.7744)
  line L84 (9.7535, 2.7744) -> (8.4032, 2.7744)
  line L85 (8.4032, 2.7744) -> (8.4032, 8.8744)
  spline S184 degree 2 poles (9.7535, 6.4155) (9.7535, 5.9689) (10.1107, 5.5223) knots 0 0 0 1 1 1
  spline S185 degree 2 poles (10.1107, 5.5223) (10.4207, 5.3068) (10.8673, 5.3068) knots 0 0 0 1 1 1
  spline S186 degree 2 poles (10.8673, 5.3068) (11.3139, 5.3068) (11.6449, 5.6379) knots 0 0 0 1 1 1
  spline S187 degree 2 poles (11.6449, 5.6379) (11.9759, 5.9689) (11.9759, 6.4155) knots 0 0 0 1 1 1
  spline S188 degree 2 poles (11.9759, 6.4155) (11.9759, 6.8673) (11.3139, 7.5293) (10.8673, 7.5293) knots 0 0 0 1 2 2 2
  spline S189 degree 2 poles (10.8673, 7.5293) (10.4207, 7.5293) (9.7535, 6.8621) (9.7535, 6.4155) knots 0 0 0 1 2 2 2
  spline S190 degree 2 poles (10.1895, 6.4155) (10.1895, 6.6887) (10.5889, 7.088) (10.8673, 7.088) knots 0 0 0 1 2 2 2
  spline S191 degree 2 poles (10.8673, 7.088) (11.1353, 7.088) (11.5398, 6.6834) (11.5398, 6.4155) knots 0 0 0 1 2 2 2
  spline S192 degree 2 poles (11.5398, 6.4155) (11.5398, 6.1475) (11.3402, 5.9478) knots 0 0 0 1 1 1
  spline S193 degree 2 poles (11.3402, 5.9478) (11.1353, 5.7429) (10.8673, 5.7429) knots 0 0 0 1 1 1
  spline S194 degree 2 poles (10.8673, 5.7429) (10.5941, 5.7429) (10.4522, 5.9216) knots 0 0 0 1 1 1
  spline S195 degree 2 poles (10.4522, 5.9216) (10.1895, 6.1475) (10.1895, 6.4155) knots 0 0 0 1 1 1
  line L86 (3.0913, 5.3068) -> (3.7743, 5.3068)
  spline S196 degree 2 poles (3.7743, 5.3068) (4.2156, 5.3068) (4.5467, 5.6379) knots 0 0 0 1 1 1
  spline S197 degree 2 poles (4.5467, 5.6379) (4.8777, 5.9636) (4.8777, 6.4155) knots 0 0 0 1 1 1
  line L87 (4.8777, 6.4155) -> (4.8777, 8.8744)
  line L88 (4.8777, 8.8744) -> (6.228, 8.8744)
  line L89 (6.228, 8.8744) -> (6.228, 6.4155)
  spline S198 degree 2 poles (6.228, 6.4155) (6.228, 5.9689) (6.5064, 5.6641) knots 0 0 0 1 1 1
  spline S199 degree 2 poles (6.5064, 5.6641) (6.89, 5.3068) (7.3366, 5.3068) knots 0 0 0 1 1 1
  line L90 (7.3366, 5.3068) -> (8.0144, 5.3068)
  line L91 (8.0144, 5.3068) -> (8.0144, 3.9618)
  line L92 (8.0144, 3.9618) -> (7.3366, 3.9618)
  spline S200 degree 2 poles (7.3366, 3.9618) (6.2332, 3.9618) (5.5502, 4.7709) knots 0 0 0 1 1 1
  spline S201 degree 2 poles (5.5502, 4.7709) (4.8724, 3.9618) (3.7743, 3.9618) knots 0 0 0 1 1 1
  line L93 (3.7743, 3.9618) -> (3.0913, 3.9618)
  line L94 (3.0913, 3.9618) -> (3.0913, 5.3068)
  spline S202 degree 2 poles (4.8777, 3.4469) (4.8777, 3.7096) (5.2875, 4.1194) (5.5554, 4.1194) knots 0 0 0 1 2 2 2
  spline S203 degree 2 poles (5.5554, 4.1194) (5.8234, 4.1194) (6.0283, 3.9198) knots 0 0 0 1 1 1
  spline S204 degree 2 poles (6.0283, 3.9198) (6.228, 3.7149) (6.228, 3.4469) knots 0 0 0 1 1 1
  spline S205 degree 2 poles (6.228, 3.4469) (6.228, 3.1737) (6.0283, 2.974) knots 0 0 0 1 1 1
  spline S206 degree 2 poles (6.0283, 2.974) (5.8181, 2.7744) (5.5554, 2.7744) knots 0 0 0 1 1 1
  spline S207 degree 2 poles (5.5554, 2.7744) (5.2822, 2.7744) (4.8777, 3.1789) (4.8777, 3.4469) knots 0 0 0 1 2 2 2
  point P0 (28.7, 2.5)
  constraints: 2 other
extrude "Extrusion7" cut sketch "Skizze6" against normal blind 0.3
sketch "Skizze7" plane through (0, 0, 3.5) normal (0, 0, 1) x (1, 0, 0)
  circle A0 centre (37.5, -5) radius 1.5 projected
  circle A1 centre (37.5, -13) radius 1.5 projected
  circle A2 centre (37.5, -21) radius 1.5 projected
  line L0 (41.7533, -3.357) -> (46.7735, -3.357) construction
  line L1 (46.7735, -3.357) -> (46.7735, -8.1229) construction
  line L2 (46.7735, -8.1229) -> (41.7533, -8.1229) construction
  line L3 (41.7533, -8.1229) -> (41.7533, -3.357) construction
  line L4 (42.8263, 12.1985) -> (47.8465, 12.1985) construction
  line L5 (47.8465, 12.1985) -> (47.8465, 10.0309) construction
  line L6 (47.8465, 10.0309) -> (42.8263, 10.0309) construction
  line L7 (42.8263, 10.0309) -> (42.8263, 12.1985) construction
  line L8 (41.7155, -11.2777) -> (48.207, -11.2777) construction
  line L9 (48.207, -11.2777) -> (48.207, -14.8463) construction
  line L10 (48.207, -14.8463) -> (41.7155, -14.8463) construction
  line L11 (41.7155, -14.8463) -> (41.7155, -11.2777) construction
  line L12 (41.8263, -19.3419) -> (48.3177, -19.3419) construction
  line L13 (48.3177, -19.3419) -> (48.3177, -22.9904) construction
  line L14 (48.3177, -22.9904) -> (41.8263, -22.9904) construction
  line L15 (41.8263, -22.9904) -> (41.8263, -19.3419) construction
  line L16 (44.7247, -6.8656) -> (42.199, -6.8656)
  line L17 (42.199, -6.8656) -> (42.199, -3.3656)
  line L18 (42.199, -3.3656) -> (43.1018, -3.3656)
  line L19 (43.1018, -3.3656) -> (43.1018, -6.1885)
  line L20 (43.1018, -6.1885) -> (44.7247, -6.1885)
  line L21 (44.7247, -6.1885) -> (44.7247, -6.8656)
  line L22 (47.7847, -6.8656) -> (45.4476, -6.8656)
  line L23 (45.4476, -6.8656) -> (45.4476, -6.2542)
  line L24 (45.4476, -6.2542) -> (46.1847, -6.2542)
  line L25 (46.1847, -6.2542) -> (46.1847, -4.4056)
  line L26 (46.1847, -4.4056) -> (45.4476, -4.4056)
  line L27 (45.4476, -4.4056) -> (45.4476, -3.8342)
  spline S0 degree 2 poles (45.4476, -3.8342) (45.6161, -3.8342) (45.9276, -3.7942) (46.0304, -3.7456) knots 0 0 0 1 2 2 2
  spline S1 degree 2 poles (46.0304, -3.7456) (46.1533, -3.6856) (46.2733, -3.497) (46.2847, -3.357) knots 0 0 0 1 2 2 2
  line L28 (46.2847, -3.357) -> (47.0618, -3.357)
  line L29 (47.0618, -3.357) -> (47.0618, -6.2542)
  line L30 (47.0618, -6.2542) -> (47.7847, -6.2542)
  line L31 (47.7847, -6.2542) -> (47.7847, -6.8656)
  line L32 (44.687, -14.8463) -> (42.1612, -14.8463)
  line L33 (42.1612, -14.8463) -> (42.1612, -11.3463)
  line L34 (42.1612, -11.3463) -> (43.0641, -11.3463)
  line L35 (43.0641, -11.3463) -> (43.0641, -14.1691)
  line L36 (43.0641, -14.1691) -> (44.687, -14.1691)
  line L37 (44.687, -14.1691) -> (44.687, -14.8463)
  line L38 (47.9669, -14.8463) -> (45.2184, -14.8463)
  line L39 (45.2184, -14.8463) -> (45.2184, -14.2691)
  spline S2 degree 2 poles (45.2184, -14.2691) (45.5327, -14.0406) (46.1669, -13.5291) (46.3555, -13.3434) knots 0 0 0 1 2 2 2
  spline S3 degree 2 poles (46.3555, -13.3434) (46.6412, -13.0663) (46.8812, -12.6577) (46.8812, -12.4577) knots 0 0 0 1 2 2 2
  spline S4 degree 2 poles (46.8812, -12.4577) (46.8812, -12.2177) (46.5727, -11.9577) (46.2841, -11.9577) knots 0 0 0 1 2 2 2
  spline S5 degree 2 poles (46.2841, -11.9577) (46.0669, -11.9577) (45.5898, -12.1349) (45.3841, -12.2749) knots 0 0 0 1 2 2 2
  line L40 (45.3841, -12.2749) -> (45.3098, -12.2749)
  line L41 (45.3098, -12.2749) -> (45.3098, -11.4977)
  spline S6 degree 2 poles (45.3098, -11.4977) (45.4755, -11.4234) (46.1269, -11.2777) (46.4555, -11.2777) knots 0 0 0 1 2 2 2
  spline S7 degree 2 poles (46.4555, -11.2777) (47.1127, -11.2777) (47.8041, -11.8291) (47.8041, -12.3349) knots 0 0 0 1 2 2 2
  spline S8 degree 2 poles (47.8041, -12.3349) (47.8041, -12.6691) (47.4727, -13.2663) (47.1327, -13.5834) knots 0 0 0 1 2 2 2
  spline S9 degree 2 poles (47.1327, -13.5834) (46.9184, -13.7806) (46.4841, -14.112) (46.3927, -14.1777) knots 0 0 0 1 2 2 2
  line L42 (46.3927, -14.1777) -> (47.9669, -14.1777)
  line L43 (47.9669, -14.1777) -> (47.9669, -14.8463)
  line L44 (44.7977, -22.9161) -> (42.272, -22.9161)
  line L45 (42.272, -22.9161) -> (42.272, -19.4161)
  line L46 (42.272, -19.4161) -> (43.1748, -19.4161)
  line L47 (43.1748, -19.4161) -> (43.1748, -22.239)
  line L48 (43.1748, -22.239) -> (44.7977, -22.239)
  line L49 (44.7977, -22.239) -> (44.7977, -22.9161)
  spline S10 degree 2 poles (47.7348, -21.2761) (47.8491, -21.3761) (47.9863, -21.639) (47.9863, -21.8561) knots 0 0 0 1 2 2 2
  spline S11 degree 2 poles (47.9863, -21.8561) (47.9863, -22.1047) (47.792, -22.5333) (47.5891, -22.6847) knots 0 0 0 1 2 2 2
  spline S12 degree 2 poles (47.5891, -22.6847) (47.392, -22.8333) (46.8577, -22.9904) (46.4777, -22.9904) knots 0 0 0 1 2 2 2
  spline S13 degree 2 poles (46.4777, -22.9904) (46.0405, -22.9904) (45.4177, -22.8533) (45.2234, -22.7704) knots 0 0 0 1 2 2 2
  line L50 (45.2234, -22.7704) -> (45.2234, -22.0019)
  line L51 (45.2234, -22.0019) -> (45.3148, -22.0019)
  spline S14 degree 2 poles (45.3148, -22.0019) (45.5177, -22.1247) (46.0805, -22.3019) (46.312, -22.3019) knots 0 0 0 1 2 2 2
  spline S15 degree 2 poles (46.312, -22.3019) (46.4491, -22.3019) (46.7691, -22.2561) (46.8777, -22.1819) knots 0 0 0 1 2 2 2
  spline S16 degree 2 poles (46.8777, -22.1819) (46.9663, -22.1219) (47.0691, -21.9561) (47.0691, -21.799) knots 0 0 0 1 2 2 2
  spline S17 degree 2 poles (47.0691, -21.799) (47.0691, -21.6447) (46.9291, -21.479) (46.812, -21.4447) knots 0 0 0 1 2 2 2
  spline S18 degree 2 poles (46.812, -21.4447) (46.6977, -21.4047) (46.372, -21.399) (46.2348, -21.399) knots 0 0 0 1 2 2 2
  line L52 (46.2348, -21.399) -> (46.0405, -21.399)
  line L53 (46.0405, -21.399) -> (46.0405, -20.7733)
  line L54 (46.0405, -20.7733) -> (46.2405, -20.7733)
  spline S19 degree 2 poles (46.2405, -20.7733) (46.4234, -20.7733) (46.7063, -20.7504) (46.8063, -20.7076) knots 0 0 0 1 2 2 2
  spline S20 degree 2 poles (46.8063, -20.7076) (46.9091, -20.6619) (47.012, -20.5133) (47.012, -20.3704) knots 0 0 0 1 2 2 2
  spline S21 degree 2 poles (47.012, -20.3704) (47.012, -20.2619) (46.9034, -20.1333) (46.8205, -20.0961) knots 0 0 0 1 2 2 2
  spline S22 degree 2 poles (46.8205, -20.0961) (46.7291, -20.0533) (46.4805, -20.0247) (46.392, -20.0247) knots 0 0 0 1 2 2 2
  spline S23 degree 2 poles (46.392, -20.0247) (46.1691, -20.0247) (45.652, -20.179) (45.4091, -20.3219) knots 0 0 0 1 2 2 2
  line L55 (45.4091, -20.3219) -> (45.3234, -20.3219)
  line L56 (45.3234, -20.3219) -> (45.3234, -19.5619)
  spline S24 degree 2 poles (45.3234, -19.5619) (45.5177, -19.4847) (46.1805, -19.3419) (46.5205, -19.3419) knots 0 0 0 1 2 2 2
  spline S25 degree 2 poles (46.5205, -19.3419) (46.852, -19.3419) (47.352, -19.4561) (47.5148, -19.5533) knots 0 0 0 1 2 2 2
  spline S26 degree 2 poles (47.5148, -19.5533) (47.7063, -19.6704) (47.8948, -19.999) (47.8948, -20.219) knots 0 0 0 1 2 2 2
  spline S27 degree 2 poles (47.8948, -20.219) (47.8948, -20.5104) (47.532, -20.9704) (47.2348, -21.0333) knots 0 0 0 1 2 2 2
  line L57 (47.2348, -21.0333) -> (47.2348, -21.0676)
  spline S28 degree 2 poles (47.2348, -21.0676) (47.3548, -21.0847) (47.6234, -21.1819) (47.7348, -21.2761) knots 0 0 0 1 2 2 2
  point P0 (0, 0)
  constraints: 7 other
extrude "Extrusion8" cut sketch "Skizze7" against normal blind 0.6 contours L16 L17 L18 L19 L20 L21 | L22 L23 L24 L25 L26 L27 S0 S1 L28 L29 L30 L31 | L32 L33 L34 L35 L36 L37 | L38 L39 S2 S3 S4 S5 L40 L41 S6 S7 S8 S9 L42 L43 | L44 L45 L46 L47 L48 L49 | S10 S11 S12 S13 L50 L51 S14 S15 S16 S17 S18 L52 L53 L54 S19 S20 S21 S22 S23 L55 L56 S24 S25 S26 S27 L57 S28
sketch "Skizze8" plane through (-28.7, 34.2, 2.5) normal (0, 1, 0) x (1, 0, 0)
  line L0 (1.2, 15.8246) -> (80.2, 15.8246) projected
  line L1 (35.95, 15.8246) -> (45.45, 15.8246)
  line L2 (45.45, 15.8246) -> (45.45, 11.3246)
  line L3 (44.45, 10.3246) -> (36.95, 10.3246)
  line L4 (35.95, 11.3246) -> (35.95, 15.8246)
  line L5 (0, 32.5) -> (0, 0) projected
  arc A0 (44.45, 10.3246) -> (45.45, 11.3246) centre (44.45, 11.3246) ccw
  arc A1 (35.95, 11.3246) -> (36.95, 10.3246) centre (36.95, 11.3246) ccw
  line L6 (35.95, 13.5746) -> (45.45, 13.5746)
  line L7 (45.45, 13.5746) -> (45.45, 19.1782)
  line L8 (45.45, 19.1782) -> (35.95, 19.1782)
  line L9 (35.95, 19.1782) -> (35.95, 13.5746)
  point P0 (28.7, 2.5)
  point P1 (45.45, 10.3246)
  point P2 (35.95, 10.3246)
  point P3 (0, 16)
  dimension "d52" = 9.5
  dimension "d53" = 5.5
  dimension "d54" = 35.95
  dimension "d55" = 1
  dimension "d56" = 1
  constraints: 16 end point, 6 point on line, 4 parallel, 4 point on circle, 4 tangent, 2 centre point, 2 horizontal, 2 perpendicular, 1 midpoint
  measures "d52" distance of point (45.45, 10.325) point (35.95, 10.325)
  measures "d53" distance of L1.end point (45.45, 10.325)
  measures "d54" distance between parallel lines of L5 L4
  measures "d55" radius of A0
  measures "d56" radius of A1
extrude "Extrusion10" cut sketch "Skizze8" against normal blind 16.4
sketch "Skizze9" plane through (37.5, -5, -1) normal (0, 0, -1) x (-1, 0, 0)
  circle A0 centre (0, 0) radius 1.5 projected
  circle A1 centre (0, 0) radius 1.55
  circle A2 centre (0, -8) radius 1.5 projected
  circle A3 centre (0, -8) radius 1.55
  circle A4 centre (0, -16) radius 1.5 projected
  circle A5 centre (0, -16) radius 1.55
  point P0 (37.5, 5)
  dimension "d61" = 3.1
  dimension "d62" = 3.1
  dimension "d63" = 3.1
  constraints: 3 centre point, 3 coincident
  measures "d61" diameter of A1
  measures "d62" diameter of A3
  measures "d63" diameter of A5
extrude "Extrusion11" cut sketch "Skizze9" against normal blind 10 contours A0 | A2 | A4
extrude "Extrusion12" cut sketch "Skizze4" against normal up to surface (81.4 mm away) contours L0 L3 L9 L8
sketch "Skizze10" plane through (0, 0, 3.5) normal (0, 0, 1) x (1, 0, 0)
  circle A0 centre (37.5, 20) radius 3.7 projected
  circle A1 centre (37.5, 20) radius 8.5
  point P0 (0, 0)
  dimension "d71" = 17
  constraints: 1 centre point, 1 coincident
  measures "d71" diameter of A1
extrude "Extrusion13" cut sketch "Skizze10" against normal blind 1.5
